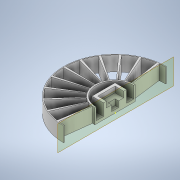
# Autodesk Inventor part: Capsule_Design_Final
Saved by Autodesk Inventor 2022 (Build 260153000, 153)
## iProperties
Created: 2023-02-21
Part Number: Capsule_Design_Final
Material: Generic
Document SubType Name: Modeling
Designer: zarek
Density: 1 g/cm^3
Appearance: Default
Author: zarek
Autodesk Inventor part; units mm, degrees
sketch "Sketch1" plane through (0, 0, 0) normal (0, 1, 0) x (-1, 0, 0)
  circle A0 centre (0, 0) radius 88.9
  dimension "d0" = 177.8
  constraints: 1 centre point, 1 coincident
  measures "d0" diameter of A0
extrude "Extrusion1" add sketch "Sketch1" along normal blind 25.4
sketch "Sketch2" plane through (0, 25.4, 0) normal (0, 1, 0) x (1, 0, 0)
  circle A0 centre (0, 0) radius 87.4
  line L0 (0, 0) -> (-10.8342, 88.2374)
  circle A1 centre (0, 0) radius 88.9 projected
  line L1 (0, 0) -> (10.8342, 88.2374)
  circle A2 centre (0, 0) radius 34.925
  line L2 (0, 0) -> (0, 88.9)
  point P0 (-4.2563, 34.6647)
  point P1 (4.2563, 34.6647)
  point P2 (10.6514, 86.7485)
  point P3 (-10.6514, 86.7485)
  dimension "d3" = 174.8
  dimension "d4" = 69.85
  dimension "d10" = 14
  dimension "d11" = 7
  constraints: 6 end point, 3 point on circle, 2 centre point, 2 coincident, 1 vertical
  measures "d3" diameter of A0
  measures "d4" diameter of A2
  measures "d10" angle of L1 L0
  measures "d11" angle of L1 L2
extrude "Extrusion2" cut sketch "Sketch2" against normal blind 25.4 contours L1 A2 L2 A0 | A0 L2 A2 L0
pattern_circular "Circular Pattern1" count 22 over 360 about axis through (0, 0, 0) along (0, 1, 0) of "Extrusion2"
sketch "Sketch4" plane through (0, 25.4, 0) normal (0, 1, 0) x (1, 0, 0)
  circle A0 centre (0, 0) radius 32.425
  dimension "d16" = 64.85
  constraints: 1 centre point, 1 coincident
  measures "d16" diameter of A0
extrude "Extrusion3" cut sketch "Sketch4" against normal blind 20.4
ref_plane "Work Plane1" through (0, 5, 0) normal (0, 1, 0) x (1, 0, 0)
sketch "Sketch5" plane through (0, 5, 0) normal (0, 1, 0) x (1, 0, 0)
  line L0 (-20, 20) -> (20, 20)
  line L1 (20, 20) -> (20, -20)
  line L2 (20, -20) -> (-20, -20)
  line L3 (-20, -20) -> (-20, 20)
  point P0 (0, 0)
  dimension "d20" = 40
  dimension "d21" = 40
  dimension "d22" = 20
  dimension "d23" = 20
  constraints: 8 end point, 2 parallel, 1 horizontal, 1 perpendicular
  measures "d20" distance between parallel lines of L2 L0
  measures "d21" distance between parallel lines of L1 L3
  measures "d22" distance from line of L3 point (0, 0)
  measures "d23" distance from line of L2 point (0, 0)
extrude "Extrusion4" add sketch "Sketch5" along normal blind 20.4
ref_plane "Work Plane2" through (0, 25.4, 0) normal (0, 1, 0) x (1, 0, 0)
sketch "Sketch6" plane through (0, 25.4, 0) normal (0, 1, 0) x (1, 0, 0)
  line L0 (-15, 15) -> (15, 15)
  line L1 (15, 15) -> (15, -15)
  line L2 (15, -15) -> (-15, -15)
  line L3 (-15, -15) -> (-15, 15)
  point P0 (0, 0)
  dimension "d26" = 30
  dimension "d27" = 15
  dimension "d28" = 15
  dimension "d29" = 30
  constraints: 8 end point, 2 parallel, 1 horizontal, 1 perpendicular
  measures "d26" distance between parallel lines of L2 L0
  measures "d27" distance from line of L2 point (0, 0)
  measures "d28" distance from line of L1 point (0, 0)
  measures "d29" distance between parallel lines of L1 L3
extrude "Extrusion5" cut sketch "Sketch6" against normal blind 10
ref_plane "Work Plane3" through (0, 15.4, 0) normal (0, 1, 0) x (1, 0, 0)
sketch "Sketch7" plane through (0, 15.4, 0) normal (0, 1, 0) x (1, 0, 0)
  line L0 (-6, 6) -> (6, 6)
  line L1 (6, 6) -> (6, -6)
  line L2 (6, -6) -> (-6, -6)
  line L3 (-6, -6) -> (-6, 6)
  line L4 (-15, 15) -> (15, 15) projected
  line L5 (15, 15) -> (15, -15) projected
  line L6 (-15, -15) -> (-15, 15) projected
  line L7 (15, -15) -> (-15, -15) projected
  point P0 (0, 0)
  dimension "d32" = 9
  dimension "d33" = 9
  dimension "d34" = 9
  dimension "d35" = 9
  constraints: 8 end point, 2 parallel, 1 horizontal, 1 perpendicular
  measures "d32" distance between parallel lines of L0 L4
  measures "d33" distance between parallel lines of L5 L1
  measures "d34" distance between parallel lines of L6 L3
  measures "d35" distance between parallel lines of L7 L2
extrude "Extrusion6" cut sketch "Sketch7" against normal blind 10 contours L0 L1 L2 L3
sketch "Sketch16" plane through (0, 0, 0) normal (0, -1, 0) x (1, 0, 0)
  point P0 (0, 0)
ref_plane "Work Plane6" through (0, 25.4, 0) normal (-1, 0, 0) x (0, 0, -1)
sketch "Sketch18" plane through (0, 25.4, 0) normal (-1, 0, 0) x (0, 0, -1)
  line L0 (-99.4236, -8.2024) -> (109.702, -8.2024)
  line L1 (109.702, -8.2024) -> (109.702, 39.2363)
  line L2 (109.702, 39.2363) -> (-99.4236, 39.2363)
  line L3 (-99.4236, 39.2363) -> (-99.4236, -8.2024)
  point P0 (0, 25.4)
  constraints: 8 end point, 2 parallel, 1 horizontal, 1 perpendicular
extrude "Extrusion7" cut sketch "Sketch18" against normal blind 127
equation "\"d11\" = 0.5 * d10"
equation "\"d21\" = d20"
equation "\"d22\" = 0.5 * d20"
equation "\"d23\" = 0.5 * d20"
equation "\"d27\" = 0.5 * d26"
equation "\"d28\" = 0.5 * d26"
equation "\"d29\" = d26"
equation "\"d33\" = d32"
equation "\"d34\" = d32"
equation "\"d35\" = d32"
body "Solid1"
